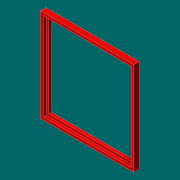
# Autodesk Inventor part: aerogelHolder
Saved by Autodesk Inventor 2016 (Build 200138000, 138)
## iProperties
Created: 2015-10-27
Part Number: aerogelHolder
Material: ABS Plastic
Document SubType Name: Modeling
Designer: Sawaiz
Density: 1.06 g/cm^3
Appearance: Smooth - Red
Author: Sawaiz
Autodesk Inventor part; units mm, degrees
ref_plane "YZ Plane" through (0, 0, 0) normal (1, 0, 0) x (0, 1, 0)
ref_plane "XZ Plane" through (0, 0, 0) normal (0, 1, 0) x (-1, 0, 0)
ref_plane "XY Plane" through (0, 0, 0) normal (0, 0, 1) x (1, 0, 0)
sketch "Sketch1" plane through (0, 0, 0) normal (1, 0, 0) x (0, 1, 0)
  line L0 (-53.975, -53.975) -> (53.975, -53.975)
  line L1 (53.975, -53.975) -> (53.975, 53.975)
  line L2 (53.975, 53.975) -> (-53.975, 53.975)
  line L3 (-53.975, 53.975) -> (-53.975, -53.975)
  line L4 (-53.975, -53.975) -> (53.975, 53.975) construction
  line L5 (53.975, -53.975) -> (-53.975, 53.975) construction
  point P0 (0, 0)
  dimension "d0" = 107.95
  dimension "d1" = 107.95
  constraints: 12 end point, 2 midpoint, 2 parallel, 1 horizontal, 1 perpendicular
  measures "d0" distance of L2.end L1.end
  measures "d1" distance of L1.end L0.end
extrude "Extrusion1" add sketch "Sketch1" along normal blind 6.35
sketch "Sketch2" plane through (6.35, 0, 0) normal (1, 0, 0) x (0, 0, -1)
  line L0 (50.8, -50.8) -> (-50.8, -50.8)
  line L1 (-50.8, -50.8) -> (-50.8, 50.8)
  line L2 (-50.8, 50.8) -> (50.8, 50.8)
  line L3 (50.8, 50.8) -> (50.8, -50.8)
  line L4 (50.8, -50.8) -> (-50.8, 50.8) construction
  line L5 (-50.8, -50.8) -> (50.8, 50.8) construction
  point P0 (0, 0)
  dimension "d4" = 101.6
  dimension "d5" = 101.6
  constraints: 12 end point, 2 midpoint, 2 parallel, 1 horizontal, 1 perpendicular
  measures "d4" distance of L1.end L2.end
  measures "d5" distance of L0.end L1.end
extrude "Extrusion2" cut sketch "Sketch2" against normal blind 3.175
sketch "Sketch3" plane through (3.175, 0, 0) normal (1, 0, 0) x (0, 0, -1)
  line L0 (50.8, -50.8) -> (-50.8, -50.8) projected
  line L1 (50.8, 50.8) -> (50.8, -50.8) projected
  line L2 (-50.8, 50.8) -> (50.8, 50.8) projected
  line L3 (-50.8, -50.8) -> (-50.8, 50.8) projected
  line L4 (-47.625, 47.625) -> (47.625, 47.625)
  line L5 (47.625, 47.625) -> (47.625, -47.625)
  line L6 (47.625, -47.625) -> (-47.625, -47.625)
  line L7 (-47.625, -47.625) -> (-47.625, 47.625)
  point P0 (0, 0)
  dimension "d8" = 3.175
  constraints: 8 end point, 3 other
  measures "d8" distance between parallel lines of L3 L7
extrude "Extrusion3" cut sketch "Sketch3" against normal through all contours L4 L5 L6 L7
equation "\"d0\" = width + internalAcrylicThickness"
equation "\"d1\" = height + internalAcrylicThickness"
equation "\"d2\" = internalAcrylicThickness"
equation "\"d4\" = aerogelHeight"
equation "\"d5\" = aerogelWidth"
equation "\"d6\" = 0.5 * internalAcrylicThickness"
equation "\"d9\" = 0.5 * internalAcrylicThickness"
equation "\"frameAcrylicThickness\" = 9.525"
equation "\"internalAcrylicThickness\" = 6.35"
equation "\"aerogelWidth\" = 101.6"
equation "\"aerogelHeight\" = 101.6"
equation "\"height\" = 101.6"
equation "\"width\" = 101.6"
equation "\"depth\" = 203.2"
equation "\"mirrorAngle\" = 5deg"
equation "\"detectorWidth\" = 52"
equation "\"detectorHeight\" = 52"
equation "\"mirrorThickness\" = 3.175"
equation "\"fresnelThickness\" = 0.1"
equation "\"focalLength\" = 76.2"
equation "\"ior\" = 1.49"
equation "\"centerThickness\" = 1.524"
equation "\"fresnelAngle\" = 90deg"
equation "\"fresnelEffectiveDiameter\" = 76.2"
equation "\"oRingWidth\" = 1.5875"
equation "\"sensorHolderDepth\" = 19.05"
body "Solid1"
